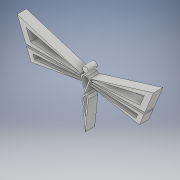
# Autodesk Inventor part: Dragonfly_logo
Saved by Autodesk Inventor 2019 (Build 230136000, 136)
## iProperties
Created: 2019-03-17
Part Number: Dragonfly_logo
Material: Generic
Document SubType Name: Modeling
Designer: cutla
Density: 1 g/cm^3
Appearance: Default
Author: cutla
Autodesk Inventor part; units mm, degrees
ref_plane "YZ Plane" through (0, 0, 0) normal (1, 0, 0) x (0, 1, 0)
ref_plane "XZ Plane" through (0, 0, 0) normal (0, 1, 0) x (-1, 0, 0)
ref_plane "XY Plane" through (0, 0, 0) normal (0, 0, 1) x (1, 0, 0)
sketch "Sketch1" plane through (0, 0, 0) normal (0, 0, 1) x (1, 0, 0)
  line L0 (0, 100) -> (0, -100) construction
  line L1 (-100, 0) -> (100, 0) construction
  circle A0 centre (0, 22) radius 3
  line L2 (-2.5, 17.2994) -> (2.5, 17.2994)
  line L3 (-2.5, 17.2994) -> (-5.2763, 14.1543)
  line L4 (-5.2763, 14.1543) -> (0, 0)
  line L5 (2.5, 17.2994) -> (5.2763, 14.1543)
  line L6 (5.2763, 14.1543) -> (0, 0)
  line L7 (-3.5567, 13.8357) -> (-1.8233, 15.7994)
  line L8 (-1.8233, 15.7994) -> (1.8233, 15.7994)
  line L9 (1.8233, 15.7994) -> (3.5567, 13.8357)
  line L10 (3.5567, 13.8357) -> (0, 4.2944)
  line L11 (0, 4.2944) -> (-3.5567, 13.8357)
  line L12 (-1.5, -1.4401) -> (1.5, -1.4401)
  line L13 (-5.2763, 14.1543) -> (0, -35.5665) construction
  line L14 (0, -35.5665) -> (5.2763, 14.1543) construction
  line L15 (-1.5, -1.4401) -> (-3.3684, -3.8243)
  line L16 (-3.3684, -3.8243) -> (0, -35.5665)
  line L17 (1.5, -1.4401) -> (3.3684, -3.8243)
  line L18 (3.3684, -3.8243) -> (0, -35.5665)
  line L19 (-1.8126, -4.2709) -> (-0.7698, -2.9401)
  line L20 (-0.7698, -2.9401) -> (0.7698, -2.9401)
  line L21 (0.7698, -2.9401) -> (1.8126, -4.2709)
  line L22 (1.8126, -4.2709) -> (0, -21.3519)
  line L23 (0, -21.3519) -> (-1.8126, -4.2709)
  line L24 (5.2763, 14.1543) -> (85.2763, 14.1543) construction
  line L25 (-74.3376, 40.7115) -> (-51.154, -16.7232) construction
  line L26 (-5.1372, 15.9918) -> (-72.7825, 36.8589)
  line L27 (-72.7825, 36.8589) -> (-63.6178, 14.1543)
  line L28 (-63.6178, 14.1543) -> (-6.0424, 14.1543)
  line L29 (-62.7458, 11.9941) -> (-5.7773, 11.9941)
  line L30 (-4.4217, 9.6563) -> (-57.9044, 0)
  line L31 (-62.7458, 11.9941) -> (-57.9044, 0)
  line L32 (-58.565, 18.3239) -> (-63.0567, 29.4515)
  line L33 (-56.0157, 8.7494) -> (-54.1442, 4.1129)
  line L34 (-63.0567, 29.4515) -> (-5.1372, 15.9918)
  line L35 (-56.0157, 8.7494) -> (-5.7773, 11.9941)
  line L36 (-54.1442, 4.1129) -> (-4.4217, 9.6563)
  line L37 (-58.565, 18.3239) -> (-6.0424, 14.1543)
  line L38 (-3.2754, 14.1543) -> (-6.0424, 14.1543) construction
  line L39 (-6.0424, 14.1543) -> (-85.2763, 14.1543) construction
  line L40 (74.3376, 40.7115) -> (51.154, -16.7232) construction
  line L41 (5.1372, 15.9918) -> (72.7825, 36.8589)
  line L42 (72.7825, 36.8589) -> (63.6178, 14.1543)
  line L43 (63.6178, 14.1543) -> (6.0424, 14.1543)
  line L44 (62.7458, 11.9941) -> (5.7773, 11.9941)
  line L45 (4.4217, 9.6563) -> (57.9044, 0)
  line L46 (62.7458, 11.9941) -> (57.9044, 0)
  line L47 (58.565, 18.3239) -> (63.0567, 29.4515)
  line L48 (56.0157, 8.7494) -> (54.1442, 4.1129)
  line L49 (63.0567, 29.4515) -> (5.1372, 15.9918)
  line L50 (56.0157, 8.7494) -> (5.7773, 11.9941)
  line L51 (54.1442, 4.1129) -> (4.4217, 9.6563)
  line L52 (58.565, 18.3239) -> (6.0424, 14.1543)
  point P0 (0, 17.2994)
  point P1 (0, -1.4401)
  point P2 (-9.4302, 14.1543)
  dimension "d51" = 5
  dimension "d52" = 22
  dimension "d53" = 1.5
  dimension "d54" = 3
  dimension "d56" = 1.5
  constraints: 106 end point, 17 symmetric about line, 14 point on line, 6 horizontal, 5 midpoint, 3 collinear, 2 vertical, 2 vertical alignment, 1 centre point, 1 perpendicular, 8 other
  measures "d51" distance of L2.start L2.end
  measures "d52" distance from line of L1 A0.centre
  measures "d53" distance between parallel lines of L3 L7
  measures "d54" distance of L12.start L12.end
  measures "d56" distance between parallel lines of L15 L19
extrude "Extrusion2" add sketch "Sketch1" along normal blind 10
body "Solid2"
